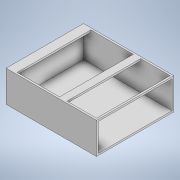
# Autodesk Inventor part: ShootingMech_Housing2
Saved by Autodesk Inventor 2020 (Build 240168000, 168)
## iProperties
Created: 2021-12-09
Part Number: ShootingMech_Housing2
Material: Generic
Document SubType Name: Modeling
Designer: danie
Density: 1 g/cm^3
Appearance: Default
Author: danie
Autodesk Inventor part; units mm, degrees
ref_plane "YZ Plane" through (0, 0, 0) normal (1, 0, 0) x (0, 1, 0)
ref_plane "XZ Plane" through (0, 0, 0) normal (0, 1, 0) x (-1, 0, 0)
ref_plane "XY Plane" through (0, 0, 0) normal (0, 0, 1) x (1, 0, 0)
sketch "Sketch1" plane through (0, 0, 0) normal (0, 1, 0) x (-1, 0, 0)
  line L0 (0, 0) -> (-152.4, 0)
  line L1 (-152.4, 0) -> (-152.4, 127)
  line L2 (-152.4, 127) -> (0, 127)
  line L3 (0, 127) -> (0, 0)
  dimension "d0" = 152.4
  dimension "d1" = 127
  constraints: 8 end point, 2 parallel, 1 horizontal, 1 perpendicular
  measures "d0" distance of L1.end L2.end
  measures "d1" distance of L0.end L1.end
extrude "Extrusion1" add sketch "Sketch1" along normal blind 3.175
sketch "Sketch2" plane through (0, 3.175, 0) normal (0, 1, 0) x (1, 0, 0)
  line L0 (152.4, 0) -> (0, 0) projected
  line L1 (0, 0) -> (3.175, 0)
  line L2 (3.175, 0) -> (3.175, -127)
  line L3 (3.175, -127) -> (0, -127)
  line L4 (0, -127) -> (0, 0)
  dimension "d4" = 3.175
  dimension "d5" = 127
  constraints: 8 end point, 2 parallel, 1 horizontal, 1 perpendicular
  measures "d4" distance of L2.end L3.end
  measures "d5" distance of L1.end L2.end
extrude "Extrusion2" add sketch "Sketch2" along normal blind 50.8
sketch "Sketch3" plane through (0, 0, 127) normal (0, 0, 1) x (1, 0, 0)
  line L0 (0, 0) -> (0, 53.975) projected
  line L1 (152.4, 0) -> (152.4, 3.175) projected
  line L2 (0, 53.975) -> (152.4, 53.975)
  line L3 (152.4, 53.975) -> (152.4, 0)
  line L4 (152.4, 0) -> (0, 0)
  line L5 (0, 0) -> (0, 53.975)
  constraints: 8 end point, 2 parallel, 1 horizontal, 1 perpendicular
extrude "Extrusion3" add sketch "Sketch3" along normal blind 3.175
sketch "Sketch4" plane through (152.4, 0, 0) normal (0, 0, -1) x (-1, 0, 0)
  line L0 (152.4, 0) -> (152.4, 53.975) projected
  line L1 (152.4, 0) -> (0, 0)
  line L2 (0, 0) -> (0, 53.975)
  line L3 (0, 53.975) -> (152.4, 53.975)
  line L4 (152.4, 53.975) -> (152.4, 0)
  constraints: 8 end point, 2 parallel, 1 horizontal, 1 perpendicular
extrude "Extrusion4" add sketch "Sketch4" along normal blind 3.175
sketch "Sketch5" plane through (152.4, 3.175, 127) normal (1, 0, 0) x (0, 0, -1)
  line L0 (-3.175, 50.8) -> (-3.175, -3.175) projected
  line L1 (-3.175, -3.175) -> (130.175, -3.175) projected
  line L2 (-3.175, 50.8) -> (130.175, 50.8)
  line L3 (130.175, 50.8) -> (130.175, -3.175)
  line L4 (130.175, -3.175) -> (-3.175, -3.175)
  line L5 (-3.175, -3.175) -> (-3.175, 50.8)
  line L6 (127, 47.625) -> (0, 47.625)
  line L7 (0, 47.625) -> (0, 0)
  line L8 (0, 0) -> (127, 0)
  line L9 (127, 0) -> (127, 47.625)
  point P0 (127, -3.175)
  dimension "d12" = 3.175
  constraints: 16 end point, 4 parallel, 2 perpendicular, 1 horizontal, 3 other
  measures "d12" distance between parallel lines of L2 L6
extrude "Extrusion5" add sketch "Sketch5" along normal blind 3.175
sketch "Sketch6" plane through (0, 53.975, 0) normal (0, 1, 0) x (1, 0, 0)
  line L0 (152.4, -127) -> (152.4, 0) construction
  line L1 (152.4, 0) -> (101.6, 0) construction
  line L2 (155.575, 0) -> (3.175, 0) construction
  line L3 (3.175, -127) -> (155.575, -127) construction
  line L4 (101.6, 0) -> (88.9, 0) construction
  line L5 (88.9, 0) -> (88.9, -127) construction
  line L6 (88.9, -127) -> (101.6, -127) construction
  line L7 (101.6, -127) -> (101.6, 0) construction
  line L8 (3.175, 0) -> (15.875, 0) construction
  line L9 (15.875, 0) -> (15.875, -127) construction
  line L10 (15.875, -127) -> (3.175, -127) construction
  line L11 (3.175, -127) -> (3.175, 0) construction
  line L12 (3.175, 0) -> (15.875, 0)
  line L13 (15.875, 0) -> (15.875, -127)
  line L14 (15.875, -127) -> (3.175, -127)
  line L15 (3.175, -127) -> (3.175, 0)
  line L16 (88.9, 0) -> (101.6, 0)
  line L17 (101.6, 0) -> (101.6, -127)
  line L18 (101.6, -127) -> (88.9, -127)
  line L19 (88.9, -127) -> (88.9, 0)
  point P0 (0, 0)
  dimension "d15" = 50.8
  dimension "d16" = 12.7
  dimension "d17" = 12.7
  constraints: 34 end point, 8 parallel, 4 horizontal, 4 perpendicular, 3 point on line
  measures "d15" distance of L0.end L1.end
  measures "d16" distance of L6.end L5.end
  measures "d17" distance of L9.end L10.end
extrude "Extrusion6" add sketch "Sketch6" against normal blind 3.175
body "Solid1"
